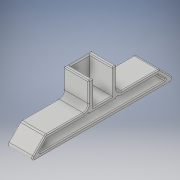
# Autodesk Inventor part: LED Stand
Saved by Autodesk Inventor 2019 (Build 230136000, 136)
## iProperties
Created: 2019-05-09
Part Number: LED Stand
Material: Generic
Document SubType Name: Modeling
Designer: Matthew XPS
Density: 1 g/cm^3
Appearance: Default
Author: Matthew XPS
Autodesk Inventor part; units mm, degrees
ref_plane "YZ Plane" through (0, 0, 0) normal (1, 0, 0) x (0, 1, 0)
ref_plane "XZ Plane" through (0, 0, 0) normal (0, 1, 0) x (-1, 0, 0)
ref_plane "XY Plane" through (0, 0, 0) normal (0, 0, 1) x (1, 0, 0)
sketch "Sketch1" plane through (0, 0, 0) normal (1, 0, 0) x (0, 1, 0)
  point P0 (0, 0)
sketch "Sketch2" plane through (0, 0, 0) normal (1, 0, 0) x (0, 1, 0)
  line L0 (0, 0) -> (0, -51.0516)
  line L1 (3.4142, -52.4658) -> (12.1142, -43.7658)
  line L2 (12.7, -42.3516) -> (12.7, -14.45)
  line L3 (12.7, 0) -> (12.7, -7.45)
  line L4 (12.7, -7.45) -> (31.75, -7.45)
  line L5 (31.75, -7.45) -> (31.75, 0)
  line L6 (0, 0) -> (12.7, 0)
  line L7 (31.75, -7.45) -> (12.7, -7.45)
  line L8 (12.7, -7.45) -> (12.7, -10.45)
  line L9 (16.7, -10.45) -> (31.75, -10.45)
  line L10 (31.75, -10.45) -> (31.75, -7.45)
  arc A0 (0, -51.0516) -> (3.4142, -52.4658) centre (2, -51.0516) ccw
  arc A1 (12.1142, -43.7658) -> (12.7, -42.3516) centre (10.7, -42.3516) ccw
  arc A2 (16.7, -10.45) -> (12.7, -14.45) centre (16.7, -14.45) ccw
  point P0 (0, -55.88)
  dimension "d0" = 55.88
  dimension "d1" = 7.45
  dimension "d2" = 19.05
  dimension "d3" = 45
  dimension "d5" = 12.7
  dimension "d6" = 3
  dimension "d7" = 2
  dimension "d8" = 4
  constraints: 22 end point, 6 point on circle, 6 point on line, 6 tangent, 3 centre point, 3 parallel, 2 horizontal, 2 perpendicular, 2 vertical, 1 equal radius
  measures "d0" distance of L0.start point (0, -55.88)
  measures "d1" distance of L3.start L3.end
  measures "d2" distance of L3.end L4.end
  measures "d3" angle of L1 L0
  measures "d5" distance of L0.start L3.start
  measures "d6" distance of L8.end L7.end
  measures "d7" radius of A0
  measures "d8" radius of A2
extrude "Extrusion1" add sketch "Sketch2" along normal blind 19.05
mirror "Mirror1" about plane through (0, 0, 0) normal (0, 0, 1) of "Extrusion1"
shell "Shell1" thickness 3 removed faces 1 at (19.05, 4.2333, -2.4833)
sketch "Sketch3" plane through (0, 0, 0) normal (-1, 0, 0) x (0, 0, 1)
  line L0 (7.45, 31.75) -> (7.45, 12.7) projected
  line L1 (-7.45, 12.7) -> (7.45, 12.7)
  line L2 (7.45, 12.7) -> (7.45, 31.75)
  line L3 (7.45, 31.75) -> (-7.45, 31.75)
  line L4 (-7.45, 31.75) -> (-7.45, 12.7)
  point P0 (0, 0)
  constraints: 8 end point, 2 parallel, 1 horizontal, 1 perpendicular
extrude "Extrusion2" add sketch "Sketch3" against normal blind 2
fillet "Fillet2" radius 0.7 4 edges at (11.025, 9.7, 10.45) (11.025, 9.7, -10.45) (11.025, 10.9554, -10.45) (11.025, 10.9554, 10.45)
fillet "Fillet3" radius 0.7 15 edges at (11.025, 9.7, 41.9374) (11.025, 3, 48.6374) (3, 3, 0) (3, 9.8859, -12.8475) (3, 10.468, -10.7876) (3, 9.8094, -10.1258) (3, 9.7, 0) (3, 9.8094, 10.1258) (3, 10.468, 10.7876) (3, 9.8859, 12.8475) (3, 9.7, 28.1937) (3, 9.7, -28.1937) (11.025, 9.7, -41.9374) (3, 6.35, -45.2874) (11.025, 3, -48.6374)
fillet "Fillet4" radius 0.7 38 edges at (9.525, 31.75, 10.45) (10.525, 31.75, 7.45) (2, 31.75, 0) (10.525, 31.75, -7.45) (9.525, 31.75, -10.45) (0, 31.75, 0) (19.05, 31.75, 8.95) (19.05, 31.75, -8.95) (19.05, 13.8716, -11.6216) (19.05, 12.7, -28.4008) (19.05, 12.5478, -43.1169) (19.05, 7.7642, -48.1158) (19.05, 1.2346, -52.8993) (19.05, 0, 0) (19.05, 1.2346, 52.8993) (19.05, 7.7642, 48.1158) (19.05, 12.5478, 43.1169) (19.05, 12.7, 28.4008) (19.05, 13.8716, 11.6216) (19.05, 24.225, 10.45) (19.05, 24.225, -10.45) (19.05, 12.7, 0) (19.05, 9.6467, -41.9153) (19.05, 6.845, -44.7924) (19.05, 3.4321, -47.5941) (19.05, 3, 0) (19.05, 3.4321, 47.5941) (19.05, 6.845, 44.7924) (19.05, 9.6467, 41.9153) (19.05, 9.7, 28.0487) (19.05, 9.8859, 12.8475) (19.05, 10.468, 10.7876) (19.05, 9.8094, 10.1258) (19.05, 9.7, 0) (19.05, 9.8094, -10.1258) (19.05, 10.468, -10.7876) (19.05, 9.8859, -12.8475) (19.05, 9.7, -28.0487)
fillet "Fillet5" radius 0.7 15 edges at (0.205, 31.545, -10.245) (0, 13.8716, -11.6216) (0, 12.7, -28.4008) (0, 12.5478, -43.1169) (0, 7.7642, -48.1158) (0, 1.2346, -52.8993) (0, 0, 0) (0, 1.2346, 52.8993) (0, 7.7642, 48.1158) (0, 12.5478, 43.1169) (0, 12.7, 28.4008) (0, 13.8716, 11.6216) (0, 23.875, 10.45) (0.205, 31.545, 10.245) (0, 23.875, -10.45)
body "Solid1"
